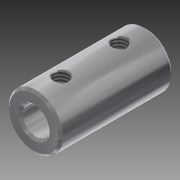
# Autodesk Inventor part: 739276_Body
Saved by Autodesk Inventor 2018 (Build 220112000, 112)
## iProperties
Category: Fasteners
Company: Autodesk Inc.
Created: 2014-11-27
Part Number: 739276_Body
Material: Aluminum 6061
Document SubType Name: Modeling
Designer: Tetrix
Density: 2.7 g/cm^3
Appearance: Aluminum - Polished
Catalog Web Link: http://www.tetrixrobotics.com/TETRIX_Motor-Axle_Shaft_Couplers
Vendor: Tetrix
Mass: 5.89159 g
Surface Area: 15.5781 cm^2
Volume: 2.18207 cm^3
Author: Autodesk Inc.
Autodesk Inventor part; units mm, degrees
ref_plane "YZ Plane" through (0, 0, 0) normal (1, 0, 0) x (0, 1, 0)
ref_plane "XZ Plane" through (0, 0, 0) normal (0, 1, 0) x (-1, 0, 0)
sketch "Sketch1" plane through (0, 0, 0) normal (0, 1, 0) x (-1, 0, 0)
  circle A0 centre (0, 0) radius 6
  dimension "d0" = 12
  constraints: 1 centre point, 1 coincident
  measures "d0" diameter of A0
extrude "Extrusion1" add sketch "Sketch1" against normal blind 25
sketch "Sketch2" plane through (0, -25, 0) normal (0, -1, 0) x (1, 0, 0)
  point P0 (0, 0)
hole "Hole1" at (0, -25, 0) direction (0, 1, 0) diameter 4.75 end through all
chamfer "Chamfer1" distance 0.5 angle 45 4 edges at (6, -25, 0) (6, 0, 0) (0, -25, 2.375) (0, 0, 2.375)
ref_plane "Work Plane1" through (0, 0, 6) normal (0, 0, 1) x (1, 0, 0)
sketch "Sketch3" plane through (0, 0, 6) normal (0, 0, 1) x (1, 0, 0)
  line L0 (5.5, -25) -> (-5.5, -25) projected
  line L1 (-2.875, -25) -> (2.875, -25) projected
  line L2 (0, -30) -> (0, 5) projected
  line L3 (-5.5, 0) -> (5.5, 0) projected
  point P0 (0, 0)
  point P1 (0, -19)
  point P2 (0, -6)
  dimension "d13" = 6
  dimension "d14" = 6
  constraints: 2 point on line
  measures "d13" distance from line of point (0, -19) L0
  measures "d14" distance from line of point (0, -6) L3
hole "Hole2" at (0, -19, 6) at (0, -6, 6) direction (0, 0, -1) diameter 3.242 end up to surface thread size "M4x0.7" class "6H" standard "ANSI Metric M Profile"
chamfer "Chamfer2" distance 0.2 angle 45 4 edges at (1.6148, -18.8581, 5.7786) (-1.621, -19.0021, 5.7769) (1.6148, -5.8581, 5.7786) (-1.621, -6.0021, 5.7769)
sketch "Sketch4" plane through (0, -25, 0) normal (0, -1, 0) x (1, 0, 0)
  circle A0 centre (0, 0) radius 3
  dimension "d25" = 6
  constraints: 1 centre point, 1 coincident
  measures "d25" diameter of A0
extrude "Extrusion2" cut sketch "Sketch4" against normal blind 12.5
chamfer "Chamfer3" distance 0.5 angle 45 1 edges at (-3, -25, 0)
body "Solid1"
